reframe (Autodesk Fusion 360 design; units mm, degrees)
Autodesk Fusion 360 part; units mm, degrees
sketch "base" plane through (0, 0, 0) normal (0, 0, 1) x (1, 0, 0)
  line L0 (0, 0) -> (101, 0)
  line L1 (101, 0) -> (101, 68)
  line L2 (101, 68) -> (0, 68)
  line L3 (0, 68) -> (0, 0)
  line L4 (6, 6) -> (95, 6)
  line L5 (95, 6) -> (95, 62)
  line L6 (95, 62) -> (6, 62)
  line L7 (6, 62) -> (6, 6)
  line L8 (-3.5, -3.5) -> (104.5, -3.5)
  line L9 (104.5, -3.5) -> (104.5, 71.5)
  line L10 (104.5, 71.5) -> (-3.5, 71.5)
  line L11 (-3.5, 71.5) -> (-3.5, -3.5)
  line L12 (-1.75, -1.75) -> (102.75, -1.75)
  line L13 (102.75, -1.75) -> (102.75, 69.75)
  line L14 (102.75, 69.75) -> (-1.75, 69.75)
  line L15 (-1.75, 69.75) -> (-1.75, -1.75)
  line L16 (101, 68) -> (97.5, 68) construction
  line L17 (97.5, 68) -> (97.5, 64.5) construction
  line L18 (97.5, 64.5) -> (101, 64.5) construction
  line L19 (101, 64.5) -> (101, 68) construction
  circle A0 centre (97.5, 64.5) radius 3.3
  line L20 (101, 34) -> (6, 34) construction
  line L21 (101, 68) -> (50.5, 68)
  line L22 (50.5, 68) -> (50.5, 6) construction
  circle A1 centre (3.5, 64.5) radius 3.3
  circle A2 centre (3.5, 3.5) radius 3.3
  circle A3 centre (97.5, 3.5) radius 3.3
  line L23 (101, 34) -> (95, 34) construction
  line L24 (95, 34) -> (95, 49) construction
  line L25 (95, 49) -> (101, 49)
  line L26 (101, 49) -> (101, 34) construction
  line L27 (95, 19) -> (101, 19)
  line L28 (101, 68) -> (89.5, 68) construction
  line L29 (89.5, 68) -> (89.5, 62)
  line L30 (31.5, 68) -> (31.5, 62)
  dimension "displayWidth" = 101
  dimension "displayHeight" = 68
  dimension "displayBezel" = -6
  dimension "wallThickness" = 3.5
  dimension "d210" = 1.75
  dimension "d336" = 3.5
  dimension "d337" = 3.5
  dimension "screwDiameter" = 6.6
  dimension "d339" = 15
  dimension "d345" = 58
  dimension "d351" = 31.5
  constraint horizontal L0
  constraint vertical L1
  constraint horizontal L2
  constraint vertical L3
  constraint coincident L0.start L3.end
  constraint horizontal L16
  constraint vertical L17
  constraint horizontal L18
  constraint vertical L19
  constraint coincident L17.end L18.start
  constraint midpoint L1 L20.start
  constraint midpoint L7 L20.end
  constraint midpoint L2 L21.end
  constraint midpoint L4 L22.end
  constraint symmetric A0 L22 A1
  constraint symmetric A0 L20 A3
  constraint symmetric L20 A1 A2
  constraint horizontal L23
  constraint vertical L24
  constraint horizontal L25
  constraint vertical L26
  constraint symmetric L24.end L23 L27.start
  constraint symmetric L25.end L23 L27.end
  constraint perpendicular L1 L28
  constraint coincident L6 L29.end
  constraint perpendicular L6 L29
  constraint coincident L6 L30.end
  constraint perpendicular L6 L30
  constraint coincident L2 L30.start
  measures "displayWidth" distance of L0.start L0.end
  measures "displayHeight" distance of L0.start L2.end
  measures "d336" distance of L1.end L16.end
  measures "d337" distance of L1.end L18.end
  measures "screwDiameter" diameter of A0
  measures "d339" distance of L20.start L25.end
  measures "d351" distance of L3 L30.end
extrude "Extrude5" add sketch "base" along normal blind 4 from surface at 4.8 contours L0 L1 L2 L3 L4 L5 L6 L7 L27 L30 | L1 L5 L25 L27 | L2 L6 L21 L29 L30 | L1 L2 L5 L6 L21 L25 L29 | A0 | A1 | A2 | A3 makes body 1
extrude "Extrude15" cut sketch "base" along normal blind 1.1 from surface at 4.8 contours L1 L5 L25 L27 | L2 L6 L21 L29 L30 bodies 1
extrude "Extrude6" add sketch "base" along normal blind 30 contours L8 L9 L10 L11 | L12 L13 L14 L15 bodies 1
extrude "Extrude13" cut sketch "base" against normal blind 1 from surface at 30 contours L12 L13 L14 L15 bodies 1
extrude "Extrude7" add sketch "base" against normal blind 1 from surface at 30 separate body contours L0 L1 L2 L3 L4 L5 L6 L7 L27 L30 | L1 L5 L25 L27 | L2 L6 L21 L29 L30 | L1 L2 L5 L6 L21 L25 L29 | L4 L5 L6 L7 | L12 L13 L14 L15 | A0 | A1 | A2 | A3 makes body 2
move_face "OffsetFaces3" offset -0.2 4 faces at (33.6667, 0, 1.6) (0, 45.3333, 1.6) (63.5, 68, 1.6) (101, 29, 1.6) on bodies 1
hole "Hole3" at (97.5, 64.5, 0) at (97.5, 3.5, 0) at (3.5, 64.5, 0) at (3.5, 3.5, 0) direction (0, 0, 1) diameter 2.7 depth 8.8 tip angle 180 counterbore diameter 6.6 counterbore depth 7.8 bodies 1
sketch "lid lip" plane through (0, 0, 29) normal (0, 0, 1) x (-1, 0, 0)
  line L0 (0, 0) -> (0, -68)
  line L1 (0, -68) -> (-101, -68)
  line L2 (-101, -68) -> (-101, 0)
  line L3 (-101, 0) -> (0, 0)
  line L4 (1.75, -69.75) -> (1.75, 1.75)
  line L5 (1.75, 1.75) -> (-102.75, 1.75)
  line L6 (-102.75, 1.75) -> (-102.75, -69.75)
  line L7 (-102.75, -69.75) -> (1.75, -69.75)
  line L8 (0, 0) -> (-50.5, 0)
  line L9 (-101.365, -0.365) -> (-0.365, -0.365)
  line L10 (-0.365, -0.365) -> (-0.365, -68.4)
  line L11 (-101.365, -68.4) -> (-101.365, -0.365)
  line L12 (-100, -1) -> (-1, -1)
  line L13 (-1, -1) -> (-1, -67)
  line L14 (-1, -67) -> (-100, -67)
  line L15 (-100, -67) -> (-100, -1)
  line L16 (-50.5, 0) -> (-50.5, -69.75)
  line L17 (-101, -68) -> (-101, -34)
  line L18 (-101, -34) -> (0, -34)
  point P0 (-50.5, -68)
  dimension "d295" = 1
  constraint coincident L0.start L3.end
  constraint midpoint L3 L8.end
  constraint midpoint L7 L16.end
  constraint midpoint L1 P0
  constraint coincident L1.end L2.start
  constraint midpoint L2 L17.end
  constraint midpoint L0 L18.end
extrude "Extrude14" add sketch "lid lip" against normal blind 1 contours L0 L3 L8 L9 L10 L16 L18 | L0 L1 L10 L18 | L2 L3 L9 L16 | L9 L10 L12 L13 L16 L18 | L1 L10 L13 L14 L16 L18 | L2 L9 L12 L15 L16 L18 | L1 L2 L14 L15 L16 L17 L18 bodies 2
move_face "OffsetFaces12" [suppressed]
sketch "camera cutout" plane through (0, 0, 30) normal (0, 0, 1) x (-1, 0, 0)
  line L0 (2, -70.6) -> (-103.3, 2) construction
  line L1 (2, 2) -> (-103.3, -70.6) construction
  line L2 (-45.25, -28.9) -> (-56.05, -28.9)
  line L3 (-56.05, -28.9) -> (-56.05, -39.7)
  line L4 (-56.05, -39.7) -> (-45.25, -39.7)
  line L5 (-45.25, -39.7) -> (-45.25, -28.9)
  line L6 (-45.25, -28.9) -> (-56.05, -39.7) construction
  line L7 (-56.05, -28.9) -> (-45.25, -39.7) construction
  line L8 (-45.25, -39.7) -> (-56.05, -39.7)
  line L9 (-56.05, -39.7) -> (-56.05, -47)
  line L10 (-56.05, -47) -> (-45.25, -47)
  line L11 (-45.25, -47) -> (-45.25, -39.7)
  line L12 (-50.65, -34.3) -> (-50.65, -48.7) construction
  line L13 (-50.65, -48.7) -> (-38.15, -48.7) construction
  line L14 (-38.15, -48.7) -> (-63.15, -48.7)
  line L15 (-63.15, -48.7) -> (-63.15, -24.838)
  line L16 (-63.15, -24.838) -> (-38.15, -24.838)
  line L17 (-38.15, -24.838) -> (-38.15, -48.7)
  line L18 (-38.15, -48.7) -> (-40.15, -48.7) construction
  line L19 (-40.15, -48.7) -> (-40.15, -46.7) construction
  circle A0 centre (-40.15, -46.7) radius 1.1
  line L20 (-40.15, -48.7) -> (-40.15, -34.2) construction
  circle A1 centre (-40.15, -34.2) radius 1.1
  circle A2 centre (-61.15, -46.7) radius 1.1
  circle A3 centre (-61.15, -34.2) radius 1.1
  line L21 (2, -70.6) -> (2, 2)
  line L22 (2, 2) -> (-103.3, 2)
  line L23 (-103.3, 2) -> (-103.3, -70.6)
  line L24 (-103.3, -70.6) -> (2, -70.6)
  line L25 (-102.3, 1) -> (1, 1)
  line L26 (1, 1) -> (1, -69.6)
  line L27 (1, -69.6) -> (-102.3, -69.6)
  line L28 (-102.3, -69.6) -> (-102.3, 1)
  line L29 (1.75, -69.75) -> (1.75, 1.75)
  line L30 (1.75, 1.75) -> (-102.75, 1.75)
  line L31 (-102.75, 1.75) -> (-102.75, -69.75)
  line L32 (-102.75, -69.75) -> (1.75, -69.75)
  point P0 (-50.65, -34.3)
  dimension "d23" = 10.8
  dimension "d24" = 10.8
  dimension "d25" = 10.8
  dimension "d26" = 7.3
  dimension "d27" = 14.4
  dimension "d28" = 12.5
  dimension "d29" = 25
  dimension "d30" = 23.862
  dimension "d31" = 2
  dimension "d32" = 2
  dimension "d33" = 2.2
  dimension "d34" = 14.5
  dimension "d35" = 2.2
  dimension "cornerRadius" = 4.5
  constraint horizontal L2
  constraint perpendicular L2 L3
  constraint parallel L2 L4
  constraint parallel L3 L5
  constraint coincident L6 P0
  constraint coincident L7 P0
  constraint midpoint L0 P0
  constraint horizontal L8
  constraint vertical L9
  constraint horizontal L10
  constraint vertical L11
  constraint coincident P0 L12.start
  constraint perpendicular L10 L12
  constraint perpendicular L12 L13
  constraint horizontal L14
  constraint vertical L15
  constraint horizontal L16
  constraint vertical L17
  constraint perpendicular L17 L18
  constraint perpendicular L14 L19
  constraint coincident L19.end A0.centre
  constraint perpendicular L18 L20
  constraint coincident L20.end A1.centre
  constraint symmetric L12 A0 A2
  constraint symmetric L12 A1 A3
  measures "d23" distance of L3.end L4.end
  measures "d24" distance of L2.end L3.end
  measures "d25" distance of L4.end L3.end
  measures "d26" distance of L4.end L10.end
  measures "d27" distance of P0 L12.end
  measures "d28" distance of L12.end L13.end
  measures "d29" distance of L13.end L14.end
  measures "d30" distance of L13.end L16.end
  measures "d31" distance of L13.end L18.end
  measures "d32" distance of L18.end L19.end
  measures "d33" diameter of A0
  measures "d34" distance of L18.end L20.end
  measures "d35" diameter of A1
hole "Hole1" at (40.15, 34.2, 30) at (40.15, 46.7, 30) at (61.15, 46.7, 30) at (61.15, 34.2, 30) direction (0, 0, -1) diameter 2.3 end through all bodies 2 1
extrude "Extrude8" cut sketch "camera cutout" against normal blind 4 contours L2 L3 L4 L5 L8 | L4 L8 L9 L10 L11 bodies 2 1
extrude "Extrude16" cut sketch "camera cutout" along normal blind 0.5 from surface at -1 contours L14 L15 L16 L17 bodies 2
sketch "front screws" plane through (0, 0, 30) normal (0, 0, 1) x (-1, 0, 0)
  line L0 (-102.75, -69.75) -> (1.75, -69.75)
  line L1 (1.75, -69.75) -> (1.75, 1.75)
  line L2 (1.75, 1.75) -> (-102.75, 1.75)
  line L3 (-102.75, 1.75) -> (-102.75, -69.75)
  line L4 (-56.05, -28.9) -> (-45.25, -28.9)
  line L5 (-45.25, -28.9) -> (-45.25, -47)
  line L6 (-45.25, -47) -> (-56.05, -47)
  line L7 (-56.05, -47) -> (-56.05, -28.9)
  circle A0 centre (-61.15, -46.7) radius 1.15
  circle A1 centre (-40.15, -34.2) radius 1.15
  circle A2 centre (-40.15, -46.7) radius 1.15
  circle A3 centre (-61.15, -34.2) radius 1.15
  point P0 (-3.5, -3.5)
  point P1 (-97.5, -3.5)
  point P2 (-97.5, -64.5)
  point P3 (-3.5, -64.5)
hole "Hole2" at (97.5, 3.5, 30) at (3.5, 3.5, 30) at (3.5, 64.5, 30) at (97.5, 64.5, 30) direction (0, 0, -1) diameter 2.7 depth 3 tip angle 180 bodies 2
sketch "ring" plane through (0, 0, 30) normal (0, 0, 1) x (-1, 0, 0)
  circle A0 centre (-50.65, -34.3) radius 25
  circle A1 centre (-50.65, -34.3) radius 8
  line L0 (-45.25, -39.7) -> (-56.05, -39.7)
  line L1 (-45.25, -39.7) -> (-45.25, -28.9)
  line L2 (-45.25, -28.9) -> (-56.05, -28.9)
  line L3 (-56.05, -28.9) -> (-56.05, -39.7)
  point P0 (-50.65, -34.3)
  dimension "d438" = 50
  dimension "d439" = 16
  constraint coincident P0 A0.centre
  measures "d438" diameter of A0
  measures "d439" diameter of A1
extrude "Extrude20" add sketch "ring" along normal blind 7 separate body contours A0 makes body 3
extrude "Extrude21" cut sketch "camera cutout" along normal blind 2 contours L4 L8 L9 L10 L11 bodies 3
extrude "Extrude22" add sketch "ring" along normal blind 2.5 from surface at 2 contours A1 bodies 3
hole "Hole6" at (40.15, 34.2, 30) at (61.15, 34.2, 30) at (61.15, 46.7, 30) at (40.15, 46.7, 30) direction (0, 0, 1) diameter 2.3 depth 4 tip angle 180 bodies 3
fillet "Fillet11" radius 7 1 edges at (73.9582, 43.3404, 37) on bodies 3
draft "Draft1" angle 70 neutral plane through (0, 0, 34.5) pull (0, 0, 1) 1 faces at (42.6898, 35.0965, 35.3333) on bodies 3
move_face "OffsetFaces4" offset -0.2 4 faces at (45.25, 40.9667, 29.8333) (48.85, 28.9, 29.8333) (56.05, 34.9333, 29.8333) (52.45, 47, 29.8333) on bodies 2
move_face "OffsetFaces5" offset -0.2 4 faces at (54.8167, 24.838, 29.1667) (38.15, 32.792, 29.1667) (46.4833, 48.7, 29.3333) (63.15, 40.746, 29.1667) on bodies 2
move_face "OffsetFaces8" offset -0.2 4 faces at (45.25, 36.1, 32.8333) (48.85, 39.7, 32.8333) (48.85, 28.9, 32.8333) (56.05, 32.5, 33.6667) on bodies 3
move_face "OffsetFaces9" offset -0.2 3 faces at (45.25, 42.4684, 31.3333) (48.85, 47, 31.3333) (56.05, 42.4684, 30.6667) on bodies 3
fillet "Fillet4" radius 0.75 1 edges at (63.35, 48.9, 29.25) on bodies 2
fillet "Fillet4" radius 0.75 1 edges at (37.95, 24.638, 29.25) on bodies 2
fillet "Fillet4" radius 0.75 1 edges at (37.95, 48.9, 29.25) on bodies 2
fillet "Fillet4" radius 0.75 1 edges at (63.35, 24.638, 29.25) on bodies 2
sketch "button hole" plane through (0, 71.5, 0) normal (0, 1, 0) x (-1, 0, 0)
  line L0 (-104.5, 0) -> (3.5, 0)
  line L1 (3.5, 0) -> (3.5, 30)
  line L2 (3.5, 30) -> (-104.5, 30)
  line L3 (-104.5, 30) -> (-104.5, 0)
  circle A0 centre (-14, 17) radius 6 construction
  dimension "d419" = 17
  measures "d419" distance of L0 A0.centre
hole "Hole4" at (14, 71.5, 17) direction (0, -1, 0) diameter 12.2 depth 10 tip angle 180 counterbore diameter 14.5 counterbore depth 2 bodies 1
fillet "Fillet7" radius 0.75 1 edges at (16.6217, 71.5, 10.2406) on bodies 1
sketch "usb c hole" plane through (-3.5, 0, 0) normal (-1, 0, 0) x (0, -1, 0)
  line L0 (-71.5, 0) -> (3.5, 0)
  line L1 (3.5, 0) -> (3.5, 30)
  line L2 (3.5, 30) -> (-71.5, 30)
  line L3 (-71.5, 30) -> (-71.5, 0)
  line L4 (3.5, 15) -> (-71.5, 15) construction
  line L5 (-37.25, 16.95) -> (-30.75, 16.95)
  line L6 (-29.25, 15.45) -> (-29.25, 14.55)
  line L7 (-30.75, 13.05) -> (-37.25, 13.05)
  line L8 (-38.75, 14.55) -> (-38.75, 15.45)
  line L9 (-38.75, 16.95) -> (-29.25, 13.05) construction
  line L10 (-29.25, 16.95) -> (-38.75, 13.05) construction
  arc A0 (-29.25, 15.45) -> (-30.75, 16.95) centre (-30.75, 15.45) ccw
  arc A1 (-30.75, 13.05) -> (-29.25, 14.55) centre (-30.75, 14.55) ccw
  arc A2 (-38.75, 14.55) -> (-37.25, 13.05) centre (-37.25, 14.55) ccw
  arc A3 (-37.25, 16.95) -> (-38.75, 15.45) centre (-37.25, 15.45) ccw
  point P0 (3.5, 15)
  point P1 (-34, 15)
  point P2 (-34, 15)
  dimension "d394" = 9.5
  dimension "d395" = 3.9
  dimension "d396" = 1.5
  dimension "d397" = 1.5
  dimension "d398" = 1.5
  dimension "d399" = 1.5
  constraint midpoint L1 P0
  constraint coincident P0 L4.start
  constraint midpoint L3 L4.end
  constraint midpoint L4 P2
  constraint horizontal L5
  constraint perpendicular L5 L6
  constraint parallel L5 L7
  constraint parallel L6 L8
  constraint coincident L9 P2
  constraint coincident L10 P2
  constraint coincident P2 P1
  constraint coincident L10.start L6
  constraint coincident L10.start L5
  constraint tangent L6 A0
  constraint tangent L5 A0
  constraint coincident L9.end L7
  constraint coincident L9.end L6
  constraint tangent L7 A1
  constraint tangent L6 A1
  constraint coincident L10.end L7
  constraint coincident L10.end L8
  constraint tangent L7 A2
  constraint tangent L8 A2
  constraint coincident L9.start L5
  constraint coincident L9.start L8
  constraint tangent L5 A3
  constraint tangent L8 A3
  measures "d394" distance of L9.end L10.end
  measures "d395" distance of L10.start L9.end
  measures "d396" radius of A0
  measures "d397" radius of A1
  measures "d398" radius of A2
  measures "d399" radius of A3
extrude "Extrude17" cut sketch "usb c hole" against normal blind 3.5 contours L5 L6 L7 L8 A0 A1 A2 A3 bodies 1
move_face "OffsetFaces13" offset -0.1 8 faces at (-1.1667, 38.4719, 16.3201) (-2.3333, 38.75, 14.85) (-1.1667, 38.2851, 13.4644) (-2.3333, 35.0833, 16.95) (-2.3333, 32.9167, 13.05) (-1.1667, 29.8228, 13.3709) (-2.3333, 29.25, 15.15) (-1.1667, 30.4661, 16.9229) on bodies 1
sketch "usb c board cutout" plane through (0, 0, 8.8) normal (0, 0, 1) x (-1, 0, 0)
  circle A0 centre (-3.5, -64.5) radius 1.35
  circle A1 centre (-97.5, -64.5) radius 1.35
  circle A2 centre (-97.5, -3.5) radius 1.35
  circle A3 centre (-3.5, -3.5) radius 1.35
  line L0 (-6, -6) -> (-6, -62)
  line L1 (-6, -62) -> (-95, -62)
  line L2 (-95, -62) -> (-95, -6)
  line L3 (-95, -6) -> (-6, -6)
  line L4 (-101, -68) -> (0, -68)
  line L5 (0, -68) -> (0, 0)
  line L6 (0, 0) -> (-101, 0)
  line L7 (-101, 0) -> (-101, -68)
  line L8 (0, -68) -> (0, 0) construction
  line L9 (0, -23.2) -> (0, -44.8) construction
  line L10 (0, -23.2) -> (-2.5, -23.2) construction
  line L11 (-2.5, -23.2) -> (-2.5, -25.7) construction
  line L12 (-2.5, -25.7) -> (0, -25.7) construction
  line L13 (0, -25.7) -> (0, -23.2) construction
  circle A4 centre (-2.5, -25.7) radius 1.5 construction
  line L14 (0, -34) -> (-13.5, -34) construction
  line L15 (0, -23.2) -> (0, -21.2)
  line L16 (0, -46.8) -> (0, -21.2)
  line L17 (0, -44.8) -> (-2.5, -44.8) construction
  line L18 (-2.5, -44.8) -> (-2.5, -42.3) construction
  line L19 (-2.5, -42.3) -> (0, -42.3) construction
  line L20 (0, -42.3) -> (0, -44.8) construction
  circle A5 centre (-2.5, -42.3) radius 1.5 construction
  line L21 (0, -44.8) -> (-6, -44.8)
  line L22 (0, -23.2) -> (-6, -23.2)
  line L23 (-6, -44.8) -> (-6, -23.2) construction
  line L24 (-6, -46.8) -> (0, -46.8)
  line L25 (0, -46.8) -> (0, -21.2)
  line L26 (0, -21.2) -> (-6, -21.2)
  line L27 (-6, -21.2) -> (-6, -46.8)
  line L28 (-6, -46.8) -> (0, -21.2) construction
  line L29 (0, -46.8) -> (-6, -21.2) construction
  point P0 (0, -34)
  point P1 (-3, -34)
  dimension "d402" = 68
  dimension "d403" = 21.6
  dimension "d404" = 2.5
  dimension "d405" = 2.5
  dimension "d406" = 3
  dimension "d407" = 13.5
  dimension "d410" = 2.5
  dimension "d411" = 2.5
  dimension "d412" = 3
  dimension "d421" = 25.6
  constraint vertical L8
  constraint coincident L4.end L5.start
  constraint midpoint L5 P0
  constraint coincident L5 L9.start
  constraint parallel L5 L9
  constraint midpoint P0 L9
  constraint horizontal L10
  constraint vertical L11
  constraint horizontal L12
  constraint vertical L13
  constraint coincident L11.end L12.start
  constraint horizontal L14
  constraint coincident P0 L14.start
  constraint perpendicular L10 L15
  constraint vertical L16
  constraint horizontal L17
  constraint vertical L18
  constraint horizontal L19
  constraint vertical L20
  constraint coincident L18.end L19.start
  constraint coincident L0 L22.end
  constraint perpendicular L0 L22
  constraint coincident L0 L21.end
  constraint perpendicular L0 L21
  constraint horizontal L24
  constraint perpendicular L24 L25
  constraint parallel L24 L26
  constraint parallel L25 L27
  constraint coincident L28 P1
  constraint coincident L29 P1
  constraint coincident L0 L24.start
  constraint coincident L14 P1
  constraint collinear L9 L25
  measures "d402" distance of L4.end L5.end
  measures "d403" distance of L9.start L9.end
  measures "d404" distance of L9.start L10.end
  measures "d405" distance of L9.start L12.end
  measures "d406" diameter of A4
  measures "d407" distance of P0 L14.end
  measures "d410" distance of L9.end L17.end
  measures "d411" distance of L9.end L19.end
  measures "d412" diameter of A5
  measures "d421" distance of L24.start L26.end
extrude "Extrude18" add sketch "usb c board cutout" along normal blind 3.5 contours L0 L5 L16 L21 L22 L25 L27 bodies 1
extrude "Extrude19" add sketch "usb c board cutout" along normal blind 5.2 contours L0 L5 L15 L16 L22 L25 L26 L27 | L0 L5 L16 L21 L24 L25 L27 bodies 1
extrude "Extrude23" add 1 faces at (6, 38.2667, 6.1333) along direction (1, 0, 0) blind 12 on bodies 1 bodies 1
sketch "Sketch20" plane through (18, 0, 0) normal (1, 0, 0) x (0, 1, 0)
  line L0 (6, 4.8) -> (62, 4.8)
  line L1 (62, 4.8) -> (62, 8.8)
  line L2 (62, 8.8) -> (46.8, 8.8)
  line L3 (46.8, 8.8) -> (46.8, 14)
  line L4 (46.8, 14) -> (44.8, 14)
  line L5 (44.8, 14) -> (44.8, 12.3)
  line L6 (44.8, 12.3) -> (23.2, 12.3)
  line L7 (23.2, 12.3) -> (23.2, 14)
  line L8 (23.2, 14) -> (21.2, 14)
  line L9 (21.2, 14) -> (21.2, 8.8)
  line L10 (21.2, 8.8) -> (6, 8.8)
  line L11 (6, 8.8) -> (6, 4.8)
  line L12 (62, 4.8) -> (6, 4.8)
  line L13 (6, 4.8) -> (6, 8.8)
  line L14 (6, 8.8) -> (62, 8.8)
  line L15 (62, 8.8) -> (62, 4.8)
  constraint horizontal L12
  constraint vertical L13
  constraint horizontal L14
  constraint vertical L15
  constraint coincident L10.end L11.start
  constraint coincident L0.end L1.start
extrude "Extrude28" add sketch "Sketch20" along normal blind 8.5 contours L0 L1 L2 L10 L11 L12 L13 L14 L15 bodies 1
move_face "OffsetFaces7" offset -0.6 2 faces at (12, 23.2, 13.4333) (12, 44.8, 13.4333) on bodies 1
hole "Hole5" at (2.5, 42.3, 8.8) at (2.5, 25.7, 8.8) direction (0, 0, 1) diameter 2.7 end up to surface (3.5 mm away) bodies 1
extrude "Extrude29" cut 2 faces at (2.4131, 26.0807, 8.8) (2.8976, 41.9701, 8.8) along direction (0, 0, -1) blind 2.5 on bodies 1 bodies 1
sketch "strap hole 1" plane through (-3.5, 0, 0) normal (-1, 0, 0) x (0, -1, 0)
  line L0 (-71.5, 0) -> (3.5, 0)
  line L1 (3.5, 0) -> (3.5, 30)
  line L2 (3.5, 30) -> (-71.5, 30)
  line L3 (-71.5, 30) -> (-71.5, 0)
  line L4 (-37.25, 17.05) -> (-30.75, 17.05)
  arc A0 (-29.15, 15.45) -> (-30.75, 17.05) centre (-30.75, 15.45) ccw
  line L5 (-29.15, 15.45) -> (-29.15, 14.55)
  arc A1 (-30.75, 12.95) -> (-29.15, 14.55) centre (-30.75, 14.55) ccw
  line L6 (-30.75, 12.95) -> (-37.25, 12.95)
  arc A2 (-38.85, 14.55) -> (-37.25, 12.95) centre (-37.25, 14.55) ccw
  line L7 (-38.85, 14.55) -> (-38.85, 15.45)
  arc A3 (-37.25, 17.05) -> (-38.85, 15.45) centre (-37.25, 15.45) ccw
  point P0 (-64.5, 15)
  dimension "d459" = 15
  dimension "d472" = 7
  measures "d459" distance of L0 P0
  measures "d472" distance of L3 P0
hole "Hole7" at (-3.5, 64.5, 15) direction (1, 0, 0) diameter 3 depth 3.5 tip angle 180 countersink diameter 3.5 countersink angle 60 bodies 1
sketch "bezel" plane through (0, 0, 0) normal (0, 0, 1) x (1, 0, 0)
  line L0 (104.5, 71.5) -> (-3.5, 71.5)
  line L1 (104.5, -3.5) -> (104.5, 71.5)
  line L2 (-3.5, -3.5) -> (104.5, -3.5)
  line L3 (-3.5, 71.5) -> (-3.5, -3.5)
  line L4 (4.5, 4.5) -> (96.5, 4.5)
  line L5 (96.5, 4.5) -> (96.5, 63.5)
  line L6 (96.5, 63.5) -> (4.5, 63.5)
  line L7 (4.5, 63.5) -> (4.5, 4.5)
  line L8 (103.5, 36) -> (102, 36)
  line L9 (102, 36) -> (102, 32)
  line L10 (102, 32) -> (103.5, 32)
  line L11 (103.5, 32) -> (103.5, 36)
  line L12 (103.5, 36) -> (102, 32) construction
  line L13 (102, 36) -> (103.5, 32) construction
  line L14 (103.5, 1.5) -> (103.5, 5.5)
  line L15 (103.5, 5.5) -> (102, 5.5)
  line L16 (102, 5.5) -> (102, 1.5)
  line L17 (102, 1.5) -> (103.5, 1.5)
  line L18 (-1, 1.5) -> (-1, 5.5)
  line L19 (-1, 5.5) -> (-2.5, 5.5)
  line L20 (-2.5, 5.5) -> (-2.5, 1.5)
  line L21 (-2.5, 1.5) -> (-1, 1.5)
  line L22 (-1, 32) -> (-1, 36)
  line L23 (-1, 36) -> (-2.5, 36)
  line L24 (-2.5, 36) -> (-2.5, 32)
  line L25 (-2.5, 32) -> (-1, 32)
  line L26 (103.5, 62.5) -> (103.5, 66.5)
  line L27 (103.5, 66.5) -> (102, 66.5)
  line L28 (102, 66.5) -> (102, 62.5)
  line L29 (102, 62.5) -> (103.5, 62.5)
  line L30 (-1, 62.5) -> (-1, 66.5)
  line L31 (-1, 66.5) -> (-2.5, 66.5)
  line L32 (-2.5, 66.5) -> (-2.5, 62.5)
  line L33 (-2.5, 62.5) -> (-1, 62.5)
  line L34 (48.5, 70.5) -> (52.5, 70.5)
  line L35 (52.5, 70.5) -> (52.5, 69)
  line L36 (52.5, 69) -> (48.5, 69)
  line L37 (48.5, 69) -> (48.5, 70.5)
  line L38 (48.5, 70.5) -> (52.5, 69) construction
  line L39 (52.5, 70.5) -> (48.5, 69) construction
  line L40 (1.5, 69) -> (1.5, 70.5)
  line L41 (5.5, 69) -> (1.5, 69)
  line L42 (1.5, 70.5) -> (5.5, 70.5)
  line L43 (5.5, 70.5) -> (5.5, 69)
  line L44 (95.5, 69) -> (95.5, 70.5)
  line L45 (99.5, 69) -> (95.5, 69)
  line L46 (95.5, 70.5) -> (99.5, 70.5)
  line L47 (99.5, 70.5) -> (99.5, 69)
  line L48 (1.5, -2.5) -> (1.5, -1)
  line L49 (5.5, -2.5) -> (1.5, -2.5)
  line L50 (1.5, -1) -> (5.5, -1)
  line L51 (5.5, -1) -> (5.5, -2.5)
  line L52 (48.5, -2.5) -> (48.5, -1)
  line L53 (52.5, -2.5) -> (48.5, -2.5)
  line L54 (48.5, -1) -> (52.5, -1)
  line L55 (52.5, -1) -> (52.5, -2.5)
  line L56 (95.5, -2.5) -> (95.5, -1)
  line L57 (99.5, -2.5) -> (95.5, -2.5)
  line L58 (95.5, -1) -> (99.5, -1)
  line L59 (99.5, -1) -> (99.5, -2.5)
  point P0 (102.75, 34)
  point P1 (50.5, 69.75)
  point P2 (50.5, 69.75)
  dimension "insideBezel" = -8
  dimension "d487" = 1.75
  dimension "d488" = 37.5
  dimension "d489" = 75
  dimension "d509" = 1.5
  dimension "d510" = 4
  dimension "d514" = 30.5
  dimension "d515" = 108
  dimension "d516" = 54
  dimension "d517" = 1.75
  dimension "d518" = 4
  dimension "d519" = 1.5
  dimension "d522" = 47
  constraint horizontal L8
  constraint perpendicular L8 L9
  constraint parallel L8 L10
  constraint parallel L9 L11
  constraint coincident L12 P0
  constraint coincident L13 P0
  constraint horizontal L34
  constraint perpendicular L34 L35
  constraint parallel L34 L36
  constraint parallel L35 L37
  constraint coincident L38 P2
  constraint coincident L39 P2
  constraint coincident P2 P1
  measures "d487" distance of L1 P0
  measures "d488" distance of L2 P0
  measures "d489" distance of L0.start L1.start
  measures "d509" distance of L9.end L10.end
  measures "d510" distance of L8.end L9.end
  measures "d515" distance of L0.start L0.end
  measures "d516" distance of L3 P2
  measures "d517" distance of L0 P2
  measures "d518" distance of L35.end L36.end
  measures "d519" distance of L34.end L35.end
extrude "Extrude25" add sketch "bezel" against normal blind 1.5 separate body contours L0 L1 L2 L3 | L8 L9 L10 L11 | L14 L15 L16 L17 | L18 L19 L20 L21 | L22 L23 L24 L25 | L26 L27 L28 L29 | L30 L31 L32 L33 | L34 L35 L36 L37 | L40 L41 L42 L43 | L44 L45 L46 L47 | L48 L49 L50 L51 | L52 L53 L54 L55 | L56 L57 L58 L59 makes body 4
extrude "Extrude26" add sketch "bezel" along normal blind 1 contours L8 L9 L10 L11 | L14 L15 L16 L17 | L18 L19 L20 L21 | L22 L23 L24 L25 | L26 L27 L28 L29 | L30 L31 L32 L33 | L34 L35 L36 L37 | L40 L41 L42 L43 | L44 L45 L46 L47 | L48 L49 L50 L51 | L52 L53 L54 L55 | L56 L57 L58 L59 bodies 4
extrude "Extrude27" cut sketch "bezel" along normal blind 1 contours L8 L9 L10 L11 | L14 L15 L16 L17 | L18 L19 L20 L21 | L22 L23 L24 L25 | L26 L27 L28 L29 | L30 L31 L32 L33 | L34 L35 L36 L37 | L40 L41 L42 L43 | L44 L45 L46 L47 | L48 L49 L50 L51 | L52 L53 L54 L55 | L56 L57 L58 L59 bodies 1
move_face "OffsetFaces10" offset -0.12 2 faces at (-2.5, 65.1667, 0.3333) (-1.5, 66.5, 0.3333) on bodies 1
fillet "Fillet1" radius 4.5 1 edges at (104.5, 71.5, 15) on bodies 1 4
fillet "Fillet1" radius 4.5 1 edges at (-3.5, -3.5, 15) on bodies 1 4
fillet "Fillet1" radius 4.5 1 edges at (-3.5, 71.5, 15) on bodies 1 4
fillet "Fillet1" radius 4.5 1 edges at (104.5, -3.5, 15) on bodies 1 4
fillet "Fillet1" radius 4.5 1 edges at (-3.5, 71.5, -0.75) on bodies 1 4
fillet "Fillet1" radius 4.5 1 edges at (-3.5, -3.5, -0.75) on bodies 1 4
fillet "Fillet1" radius 4.5 1 edges at (104.5, -3.5, -0.75) on bodies 1 4
fillet "Fillet1" radius 4.5 1 edges at (104.5, 71.5, -0.75) on bodies 1 4
fillet "Fillet5" [suppressed]
fillet "Fillet2" radius 2.75 1 edges at (-1.75, -1.75, 29.5) on bodies 2
fillet "Fillet2" radius 2.75 1 edges at (-1.75, 69.75, 29.5) on bodies 2
fillet "Fillet2" radius 2.75 1 edges at (102.75, -1.75, 29.5) on bodies 2
fillet "Fillet2" radius 2.75 1 edges at (102.75, 69.75, 29.5) on bodies 2
fillet "Fillet3" radius 2.75 1 edges at (-1.75, 69.75, 29.5) on bodies 1
fillet "Fillet3" radius 2.75 1 edges at (102.75, 69.75, 29.5) on bodies 1
fillet "Fillet3" radius 2.75 1 edges at (102.75, -1.75, 29.5) on bodies 1
fillet "Fillet3" radius 2.75 1 edges at (-1.75, -1.75, 29.5) on bodies 1
fillet "Fillet9" radius 3.5 8 edges at (103.182, -2.182, 30) (50.5, -3.5, 30) (-2.182, -2.182, 30) (-3.5, 34, 30) (-2.182, 70.182, 30) (50.5, 71.5, 30) (103.182, 70.182, 30) (104.5, 34, 30) on bodies 1
fillet "Fillet13" radius 0.5 1 edges at (4.5, 63.5, -0.75) on bodies 4
fillet "Fillet13" radius 0.5 1 edges at (96.5, 63.5, -0.75) on bodies 4
fillet "Fillet13" radius 0.5 1 edges at (96.5, 4.5, -0.75) on bodies 4
fillet "Fillet13" radius 0.5 1 edges at (4.5, 4.5, -0.75) on bodies 4
fillet "Fillet12" radius 3 1 faces at (65.6667, -0.8333, -1.5) on bodies 4
fillet "Fillet10" radius 0.3 8 edges at (50.5, 71.5, 0) (-2.182, 70.182, 0) (-3.5, 34, 0) (-2.182, -2.182, 0) (50.5, -3.5, 0) (103.182, -2.182, 0) (104.5, 34, 0) (103.182, 70.182, 0) on bodies 1
move_face "OffsetFaces11" offset -0.15 60 faces at (-2.62, 63.8733, 0.6667) (-1.54, 63.8733, 1) (-2.08, 62.5, 0.3333) (-1.54, 66.62, 0.3333) (2.8333, 70.5, 0.3333) (1.5, 70, 0.6667) (5.5, 70, 0.3333) (4.1667, 69, 0.3333) (4.1667, 69.5, 1) (52.5, 70, 0.3333) (49.8333, 69, 0.6667) (51.1667, 70.5, 0.6667) (48.5, 69.5, 0.3333) (51.1667, 70, 1) (98.1667, 69.5, 1) (96.8333, 70.5, 0.3333) (95.5, 70, 0.6667) (99.5, 70, 0.3333) (98.1667, 69, 0.3333) (103.5, 63.8333, 0.3333) (102.5, 62.5, 0.3333) (103.5, 33.3333, 0.3333) (103, 32, 0.6667) (103.5, 2.8333, 0.3333) (102.5, 1.5, 0.3333) (99.5, -1.5, 0.3333) (98.1667, -2.5, 0.3333) (49.8333, -2.5, 0.6667) (52.5, -1.5, 0.3333) (4.1667, -2.5, 0.3333) (5.5, -1.5, 0.3333) (4.1667, -2, 1) (-1, 2.8333, 0.3333) (-2, 1.5, 0.3333) (-1, 33.3333, 0.3333) (-1, 63.8733, 0.3333) (-2, 32, 0.3333) (-1.5, 2.8333, 1) (-1.5, 33.3333, 1) (51.1667, -1.5, 1) (103, 33.3333, 1) (103, 2.8333, 1) (98.1667, -2, 1) (103, 63.8333, 1) (102, 2.8333, 0.6667) (95.5, -1.5, 0.6667) (102, 34.6667, 0.3333) (102, 63.8333, 0.6667) (48.5, -1.5, 0.6667) (1.5, -1.5, 0.6667) (-2.5, 2.8333, 0.6667) (-2.5, 33.3333, 0.6667) (103, 66.5, 0.3333) (103, 36, 0.3333) (49.8333, -1, 0.3333) (2.8333, -1, 0.3333) (-1.5, 5.5, 0.3333) (-1.5, 36, 0.3333) (103, 5.5, 0.3333) (96.8333, -1, 0.3333) on bodies 1
equation "displayBezelHeight = 4 mm"
equation "cameraThick = 30 mm"
equation "d16 = displayBezelHeight"
equation "d18 = cameraThick"
equation "d20 = cameraThick"
equation "frontThickness = -1 mm"
equation "d23 = d24"
equation "d25 = d24"
equation "d28 = ( 25 / 2 ) * 1 mm"
equation "d51 = 1.50 mm"
equation "d53 = 0.5 * d51"
equation "d210 = wallThickness / 2"
equation "d211 = cameraThick"
equation "d319 = cornerRadius - wallThickness / 2"
equation "d321 = cornerRadius - wallThickness / 2"
equation "d323 = cornerRadius - wallThickness / 2"
equation "d325 = cornerRadius - wallThickness / 2"
equation "d327 = cornerRadius - wallThickness / 2"
equation "d329 = cornerRadius - wallThickness / 2"
equation "d331 = cornerRadius - wallThickness / 2"
equation "d333 = cornerRadius - wallThickness / 2"
equation "toleranceOffset = -0.2 mm"
equation "d336 = d337"
equation "displayBezelOffset = 4.8 mm"
equation "d352 = toleranceOffset"
equation "d355 = displayBezelOffset + displayBezelHeight - 1 mm"
equation "d356 = screwDiameter"
equation "d357 = displayBezelOffset + displayBezelHeight"
equation "d358 = toleranceOffset"
equation "d359 = frontThickness"
equation "d360 = -frontThickness / 2"
equation "d362 = toleranceOffset"
equation "d364 = d53"
equation "d366 = d53"
equation "d368 = d53"
equation "d370 = d53"
equation "d372 = cornerRadius - wallThickness"
equation "d374 = cornerRadius - wallThickness"
equation "d376 = cornerRadius - wallThickness"
equation "d378 = cornerRadius - wallThickness"
equation "d393 = d53"
equation "d397 = d396"
equation "d398 = d396"
equation "d399 = d396"
equation "d400 = -wallThickness"
equation "d402 = displayHeight"
equation "d405 = d404"
equation "d410 = d404"
equation "d411 = d404"
equation "d412 = d406"
equation "d413 = cameraThick / 2 - displayBezelOffset + displayBezel - 0.7 mm"
equation "d415 = cameraThick / 2 - displayBezelOffset + displayBezel + 1 mm"
equation "d419 = cameraThick / 2 + 2 mm"
equation "d421 = d403 + 4 mm"
equation "d427 = cornerRadius"
equation "d429 = cornerRadius"
equation "d431 = cornerRadius"
equation "d433 = cornerRadius"
equation "d435 = wallThickness"
equation "d453 = toleranceOffset"
equation "d454 = toleranceOffset"
equation "d459 = cameraThick / 2"
equation "d460 = wallThickness"
equation "d479 = cornerRadius"
equation "d481 = cornerRadius"
equation "d483 = cornerRadius"
equation "d485 = cornerRadius"
equation "d487 = wallThickness / 2"
equation "d488 = d489 / 2"
equation "d502 = cornerRadius + insideBezel / 2"
equation "d504 = cornerRadius + insideBezel / 2"
equation "d506 = cornerRadius + insideBezel / 2"
equation "d508 = cornerRadius + insideBezel / 2"
equation "d513 = -displayWidth - wallThickness"
equation "d514 = displayHeight / 2 - wallThickness"
equation "d516 = d515 / 2"
equation "d517 = wallThickness / 2"
equation "d522 = displayWidth / 2 - wallThickness"
equation "d523 = -displayHeight - wallThickness"
named bodies: "enclosure", "lid", "ring", "bezel"
